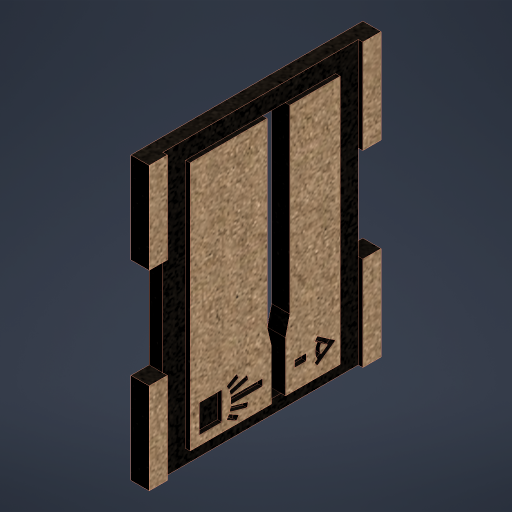
# Autodesk Inventor part: LightGate_Door_V1
Saved by Autodesk Inventor 2024.1 (Build 281209000, 209)
## iProperties
Created: 2023-05-21
Part Number: LightGate_Door_V1
Material: MDF Medium Density Fiberboard
Document SubType Name: Modeling
Designer: jaege
Density: 0.8 g/cm^3
Appearance: Red Oak - Natural Low Gloss
Mass: 15.6006 g
Surface Area: 117.953 cm^2
Volume: 19.5007 cm^3
Author: jaege
Autodesk Inventor part; units mm, degrees
ref_plane "YZ Plane" through (0, 0, 0) normal (1, 0, 0) x (0, 1, 0)
ref_plane "XZ Plane" through (0, 0, 0) normal (0, 1, 0) x (-1, 0, 0)
ref_plane "XY Plane" through (0, 0, 0) normal (0, 0, 1) x (1, 0, 0)
sketch "Sketch1" plane through (0, 0, 0) normal (1, 0, 0) x (0, 1, 0)
  line L0 (-31, -23.5) -> (-10.3333, -23.5) construction
  line L1 (31, -23.5) -> (31, 23.5)
  line L2 (31, 23.5) -> (11, 23.5)
  line L3 (-31, 23.5) -> (-31, -23.5)
  line L4 (-31, -23.5) -> (31, 23.5) construction
  line L5 (31, -23.5) -> (-31, 23.5) construction
  line L6 (-11, 23.5) -> (-11, 19.5)
  line L7 (-11, 19.5) -> (11, 19.5)
  line L8 (11, 19.5) -> (11, 23.5)
  line L9 (11, 23.5) -> (-11, 23.5) construction
  line L10 (-11, 23.5) -> (-31, 23.5)
  line L11 (31, -23.5) -> (10.3333, -23.5) construction
  line L12 (10.3333, -23.5) -> (10.3333, -27.5)
  line L13 (10.3333, -27.5) -> (31, -27.5)
  line L14 (31, -27.5) -> (31, -23.5)
  line L15 (-31, -23.5) -> (-10.3333, -23.5) construction
  line L16 (-10.3333, -23.5) -> (-10.3333, -27.5)
  line L17 (-10.3333, -27.5) -> (-31, -27.5)
  line L18 (-31, -27.5) -> (-31, -23.5)
  line L19 (10.3333, -23.5) -> (31, -23.5) construction
  line L20 (-10.3333, -23.5) -> (10.3333, -23.5)
  point P0 (0, 0)
  point P1 (11, 21.5)
  dimension "d0" = 62
  dimension "d1" = 47
  dimension "d2" = 20
  dimension "d3" = 4
  dimension "d5" = 4
  constraints: 42 end point, 13 parallel, 4 horizontal, 4 perpendicular, 3 equal length, 3 midpoint, 1 collinear, 1 horizontal alignment, 1 vertical
  measures "d0" distance of L3.start L1.end
  measures "d1" distance of L1.end L1.start
  measures "d2" distance from line of L1 point (11, 21.5)
  measures "d3" distance between parallel lines of L9 L7
  measures "d5" distance of L12.end L11.end
extrude "Outline" add sketch "Sketch1" along normal blind 4
sketch "Sketch2" plane through (4, 0, 0) normal (1, 0, 0) x (0, 0, -1)
  line L0 (3.4, 27) -> (3.4, -27.9)
  line L1 (3.4, -27.9) -> (6.5, -27.9)
  line L2 (6.5, -27.9) -> (6.5, 27)
  line L3 (6.5, 27) -> (3.4, 27)
  line L4 (-14.5, -0.45) -> (-5.55, -0.45) construction
  line L5 (-5.55, -0.45) -> (3.4, -0.45) construction
  line L6 (18.5, -0.45) -> (6.5, -0.45) construction
  line L7 (-19.5, 31) -> (23.5, 31)
  line L8 (23.5, 31) -> (23.5, -31)
  line L9 (-19.5, -31) -> (-19.5, 31)
  line L10 (-14.5, 27) -> (18.5, 27)
  line L11 (18.5, 27) -> (18.5, -27.9)
  line L12 (18.5, -27.9) -> (-14.5, -27.9)
  line L13 (-14.5, -27.9) -> (-14.5, 27)
  line L14 (-12.5, -19.7) -> (-7.5, -19.7)
  line L15 (-7.5, -19.7) -> (-7.5, -25.9)
  line L16 (-7.5, -25.9) -> (-12.5, -25.9)
  line L17 (-12.5, -25.9) -> (-12.5, -19.7)
  line L18 (-5.5, -22.05) -> (1.4, -22.05)
  line L19 (1.4, -22.05) -> (1.4, -23.55)
  line L20 (1.4, -23.55) -> (-5.5, -23.55)
  line L21 (-5.5, -23.55) -> (-5.5, -22.05)
  line L22 (13.4738, -19.9808) -> (17.5, -22.8)
  line L23 (17.5, -22.8) -> (13.4738, -25.6192)
  line L24 (13.4738, -19.9808) -> (12.9003, -20.8)
  line L25 (12.9003, -20.8) -> (15.7566, -22.8)
  line L26 (15.7566, -22.8) -> (12.9003, -24.8)
  line L27 (12.9003, -24.8) -> (13.4738, -25.6192)
  line L28 (-12.5, -22.8) -> (15.7566, -22.8) construction
  arc A0 (13.5039, -21.2227) -> (13.5039, -24.3773) centre (15.7566, -22.8) ccw
  arc A1 (14.323, -21.7962) -> (14.323, -23.8038) centre (15.7566, -22.8) ccw
  line L29 (8.5, -22.05) -> (11.0066, -22.05)
  line L30 (11.0066, -22.05) -> (11.0066, -23.55)
  line L31 (11.0066, -23.55) -> (8.5, -23.55)
  line L32 (8.5, -23.55) -> (8.5, -22.05)
  line L33 (-5.8236, -20.7956) -> (-5.548, -21.7568)
  line L34 (-5.548, -21.7568) -> (-1.703, -20.6543)
  line L35 (-1.703, -20.6543) -> (-1.9786, -19.693)
  line L36 (-1.9786, -19.693) -> (-5.8236, -20.7956)
  line L37 (-5.548, -23.8432) -> (-1.703, -24.9457)
  line L38 (-1.703, -24.9457) -> (-1.9786, -25.907)
  line L39 (-1.9786, -25.907) -> (-5.8236, -24.8044)
  line L40 (-5.8236, -24.8044) -> (-5.548, -23.8432)
  circle A2 centre (-11, -22.8) radius 5.5509 construction
  line L41 (-6.4623, -19.6028) -> (-5.9623, -20.4688)
  line L42 (-5.9623, -20.4688) -> (-3.7973, -19.2188)
  line L43 (-3.7973, -19.2188) -> (-4.2973, -18.3528)
  line L44 (-4.2973, -18.3528) -> (-6.4623, -19.6028)
  line L45 (-5.9623, -25.1312) -> (-6.4623, -25.9972)
  line L46 (-6.4623, -25.9972) -> (-4.2973, -27.2472)
  line L47 (-4.2973, -27.2472) -> (-3.7973, -26.3812)
  line L48 (-3.7973, -26.3812) -> (-5.9623, -25.1312)
  line L49 (23.5, 10.3333) -> (27.5, 10.3333) projected
  line L50 (27.5, 10.3333) -> (27.5, 31) projected
  line L51 (27.5, 31) -> (-23.5, 31) projected
  line L52 (-23.5, 31) -> (-23.5, 11) projected
  line L53 (-23.5, 11) -> (-19.5, 11) projected
  line L54 (-19.5, 11) -> (-19.5, -11) projected
  line L55 (-19.5, -11) -> (-23.5, -11) projected
  line L56 (-23.5, -11) -> (-23.5, -31) projected
  line L57 (-23.5, -31) -> (27.5, -31) projected
  line L58 (27.5, -31) -> (27.5, -10.3333) projected
  line L59 (27.5, -10.3333) -> (23.5, -10.3333) projected
  line L60 (23.5, -10.3333) -> (23.5, 10.3333) projected
  point P0 (0, 0)
  point P1 (-7.5, -22.8)
  point P2 (-5.5, -22.8)
  point P3 (13.0066, -22.8)
  point P4 (6.5, 27)
  point P5 (3.4, 27)
  dimension "d14" = 3.1
  dimension "d17" = 5
  dimension "d19" = 5
  dimension "d22" = 35
  dimension "d23" = 35
  dimension "d24" = 4
  dimension "d25" = 1
  dimension "d26" = 1
  dimension "d27" = 2.75
  dimension "d29" = 1
  dimension "d30" = 1.5
  dimension "d31" = 2
  dimension "d32" = 2
  dimension "d33" = 2
  dimension "d34" = 2
  dimension "d35" = 2
  dimension "d36" = 5
  dimension "d37" = 2
  dimension "d38" = 1
  dimension "d39" = 1
  dimension "d42" = 3.5
  dimension "d43" = 16
  dimension "d44" = 16
  dimension "d45" = 4
  dimension "d47" = 2.5
  dimension "d48" = 1
  dimension "d49" = 14
  dimension "d50" = 14
  dimension "d51" = 1
  dimension "d52" = 2.5
  dimension "d62" = 12
  dimension "d65" = 6.2
  dimension "d66" = 4
  dimension "d67" = 3.1
  constraints: 98 end point, 19 parallel, 15 perpendicular, 7 horizontal, 7 midpoint, 7 point on line, 5 point on circle, 4 collinear, 4 horizontal alignment, 3 vertical alignment, 2 centre point, 2 equal length, 1 concentric, 1 vertical, 11 other
  measures "d14" distance between parallel lines of L2 L0
  measures "d17" distance between parallel lines of L9 L13
  measures "d19" distance between parallel lines of L8 L11
  measures "d22" angle of L22 L28
  measures "d23" angle of L23 L28
  measures "d24" distance of L26.end L24.end
  measures "d25" radial gap between concentric circles of A1 A0
  measures "d26" distance between parallel lines of L22 L25
  measures "d27" radius of A0
  measures "d29" distance from line of L11 L22.end
  measures "d30" distance of L20.end L18.start
  measures "d31" distance between parallel lines of L0 L19
  measures "d32" distance between parallel lines of L2 L32
  measures "d33" distance from line of point (13.007, -22.8) L30
  measures "d34" distance between parallel lines of L13 L17
  measures "d35" distance between parallel lines of L12 L16
  measures "d36" distance between parallel lines of L17 L15
  measures "d37" distance between parallel lines of L15 L21
  measures "d38" distance of L34.end L35.end
  measures "d39" distance of L37.end L38.end
  measures "d42" distance from line of L15 point (-11, -22.8)
  measures "d43" angle of L37 L20
  measures "d44" angle of L34 L18
  measures "d45" distance of L35.end L33.start
  measures "d47" distance of L42.end L41.end
  measures "d48" distance of L42.end L43.end
  measures "d49" angle of L36 L42
  measures "d50" angle of L39 L48
  measures "d51" distance of L46.end L47.end
  measures "d52" distance of L47.end L45.start
  measures "d62" distance of L6.start L6.end
  measures "d65" distance of L16.end L14.start
  measures "d66" distance between parallel lines of L7 L10
  measures "d67" distance between parallel lines of L57 L12
extrude "Engravings" cut sketch "Sketch2" against normal blind 1 contours L3 L2 L1 L0 | L7 L8 L57 L9 | L14 L15 L16 L17 | L18 L19 L20 L21 | L22 L23 L27 L26 L25 L24 | L25 A1 L26 A0 | L29 L30 L31 L32 | L36 L35 L34 L33 | L37 L38 L39 L40 | L44 L43 L42 L41 | L48 L47 L46 L45
sketch "Sketch3" plane through (4, 0, 0) normal (1, 0, 0) x (0, 0, -1)
  line L0 (-7.5, -19.7) -> (-7.5, -25.9) projected
  line L1 (-7.5, -25.9) -> (-12.5, -25.9) projected
  line L2 (-12.5, -25.9) -> (-12.5, -19.7) projected
  line L3 (-12.5, -19.7) -> (-7.5, -19.7) projected
  line L4 (-3.7973, -26.3812) -> (-4.2973, -27.2472) projected
  line L5 (-4.2973, -27.2472) -> (-6.4623, -25.9972) projected
  line L6 (-6.4623, -25.9972) -> (-5.9623, -25.1312) projected
  line L7 (-5.9623, -25.1312) -> (-3.7973, -26.3812) projected
  line L8 (1.4, -22.05) -> (1.4, -23.55)
  line L9 (1.4, -23.55) -> (-5.5, -23.55) projected
  line L10 (-5.5, -23.55) -> (-5.5, -22.05) projected
  line L11 (-5.5, -22.05) -> (1.4, -22.05) projected
  line L12 (-4.2973, -18.3528) -> (-3.7973, -19.2188) projected
  line L13 (-3.7973, -19.2188) -> (-5.9623, -20.4688) projected
  line L14 (-5.9623, -20.4688) -> (-6.4623, -19.6028) projected
  line L15 (-6.4623, -19.6028) -> (-4.2973, -18.3528) projected
  line L16 (-1.9786, -19.693) -> (-1.703, -20.6543) projected
  line L17 (-1.703, -20.6543) -> (-5.548, -21.7568) projected
  line L18 (-5.548, -21.7568) -> (-5.8236, -20.7956) projected
  line L19 (-5.8236, -20.7956) -> (-1.9786, -19.693) projected
  line L20 (-1.703, -24.9457) -> (-1.9786, -25.907) projected
  line L21 (-1.9786, -25.907) -> (-5.8236, -24.8044) projected
  line L22 (-5.8236, -24.8044) -> (-5.548, -23.8432) projected
  line L23 (-5.548, -23.8432) -> (-1.703, -24.9457) projected
  line L24 (23.5, -31) -> (-19.5, -31) projected
  line L25 (23.5, 31) -> (23.5, 10.3333) projected
  line L26 (-19.5, 31) -> (23.5, 31) projected
  line L27 (-19.5, -11) -> (-19.5, 11) projected
  line L28 (18.5, -27.9) -> (18.5, 27) projected
  line L29 (-14.5, 27) -> (-14.5, -27.9) projected
  line L30 (3.4, -27.9) -> (6.5, -27.9)
  line L31 (2.45, 27) -> (2.45, -12.8)
  line L32 (2.45, -12.8) -> (3.4, -16.8)
  line L33 (7.45, 27) -> (7.45, -12.8)
  line L34 (7.45, -12.8) -> (6.5, -16.8)
  line L35 (6.5, -16.8) -> (6.5, -27.9)
  line L36 (-19.5, -31) -> (-19.5, -11) projected
  line L37 (23.5, 10.3333) -> (23.5, -10.3333) projected
  line L38 (-19.5, 11) -> (-19.5, 31) projected
  line L39 (23.5, -10.3333) -> (27.5, -10.3333) projected
  line L40 (27.5, -10.3333) -> (27.5, -31) projected
  line L41 (-14.5, -27.9) -> (18.5, -27.9) projected
  line L42 (3.4, -27.9) -> (3.4, 27) construction
  line L43 (6.5, 27) -> (6.5, -27.9) construction
  line L44 (18.5, 27) -> (6.5, 27) projected
  line L45 (3.4, 27) -> (-14.5, 27) projected
  line L46 (3.4, 27) -> (6.5, 27)
  line L47 (3.4, -27.9) -> (3.4, 27) construction
  line L48 (3.4, -16.8) -> (3.4, -27.9)
  point P0 (0, 0)
  dimension "d68" = 5
  dimension "d69" = 11.1
  dimension "d70" = 4
  constraints: 18 end point, 5 horizontal alignment, 2 vertical, 1 collinear, 1 equal length, 1 perpendicular, 1 vertical alignment
  measures "d68" distance between parallel lines of L33 L31
  measures "d69" distance of L34.end L30.end
  measures "d70" vertical distance of L34.end L33.end
extrude "Groove" cut sketch "Sketch3" against normal up to next contours L30 L48 L32 L31 L45 L46 L44 L33 L34 L35
sketch "Sketch4" plane through (3, 0, 0) normal (1, 0, 0) x (0, 0, -1)
  line L0 (-7.5, -25.9) -> (-7.5, -19.7) projected
  line L1 (-7.5, -19.7) -> (-12.5, -19.7) projected
  line L2 (-12.5, -19.7) -> (-12.5, -25.9) projected
  line L3 (-12.5, -25.9) -> (-7.5, -25.9) projected
  line L4 (-4.2973, -27.2472) -> (-3.7973, -26.3812) projected
  line L5 (-3.7973, -26.3812) -> (-5.9623, -25.1312) projected
  line L6 (-5.9623, -25.1312) -> (-6.4623, -25.9972) projected
  line L7 (-6.4623, -25.9972) -> (-4.2973, -27.2472) projected
  line L8 (14.323, -21.7962) -> (15.7566, -22.8) projected
  line L9 (15.7566, -22.8) -> (14.323, -23.8038) projected
  arc A0 (14.323, -21.7962) -> (14.323, -23.8038) centre (15.7566, -22.8) ccw projected
  line L10 (13.4738, -25.6192) -> (17.5, -22.8) projected
  line L11 (17.5, -22.8) -> (13.4738, -19.9808) projected
  line L12 (13.4738, -19.9808) -> (12.9003, -20.8) projected
  line L13 (12.9003, -20.8) -> (13.5039, -21.2227) projected
  arc A1 (13.5039, -21.2227) -> (13.5039, -24.3773) centre (15.7566, -22.8) ccw projected
  line L14 (13.5039, -24.3773) -> (12.9003, -24.8) projected
  line L15 (12.9003, -24.8) -> (13.4738, -25.6192) projected
  line L16 (1.4, -23.55) -> (1.4, -22.05) projected
  line L17 (1.4, -22.05) -> (-5.5, -22.05) projected
  line L18 (-5.5, -22.05) -> (-5.5, -23.55) projected
  line L19 (-5.5, -23.55) -> (1.4, -23.55) projected
  line L20 (27.5, 10.3333) -> (23.5, 10.3333) projected
  line L21 (27.5, 31) -> (27.5, 10.3333) projected
  line L22 (-23.5, 31) -> (-19.5, 31) projected
  line L23 (-19.5, -31) -> (-23.5, -31) projected
  line L24 (-23.5, 11) -> (-23.5, 31) projected
  line L25 (-19.5, 11) -> (-23.5, 11) projected
  line L26 (-23.5, -31) -> (-23.5, -11) projected
  line L27 (-23.5, -11) -> (-19.5, -11) projected
  line L28 (-3.7973, -19.2188) -> (-4.2973, -18.3528) projected
  line L29 (-4.2973, -18.3528) -> (-6.4623, -19.6028) projected
  line L30 (-6.4623, -19.6028) -> (-5.9623, -20.4688) projected
  line L31 (-5.9623, -20.4688) -> (-3.7973, -19.2188) projected
  line L32 (11.0066, -23.55) -> (11.0066, -22.05) projected
  line L33 (11.0066, -22.05) -> (8.5, -22.05) projected
  line L34 (8.5, -22.05) -> (8.5, -23.55) projected
  line L35 (8.5, -23.55) -> (11.0066, -23.55) projected
  line L36 (-1.703, -20.6543) -> (-1.9786, -19.693) projected
  line L37 (-1.9786, -19.693) -> (-5.8236, -20.7956) projected
  line L38 (-5.8236, -20.7956) -> (-5.548, -21.7568) projected
  line L39 (-5.548, -21.7568) -> (-1.703, -20.6543) projected
  line L40 (-1.9786, -25.907) -> (-1.703, -24.9457) projected
  line L41 (-1.703, -24.9457) -> (-5.548, -23.8432) projected
  line L42 (-5.548, -23.8432) -> (-5.8236, -24.8044) projected
  line L43 (-5.8236, -24.8044) -> (-1.9786, -25.907) projected
  line L44 (18.5, 27) -> (18.5, -27.9) projected
  line L45 (-14.5, -27.9) -> (-14.5, 27) projected
  line L46 (3.4, -27.9) -> (-14.5, -27.9) projected
  line L47 (23.5, -31) -> (-19.5, -31) projected
  line L48 (-19.5, -11) -> (-19.5, -31) projected
  line L49 (-19.5, -11) -> (-19.5, 11) projected
  line L50 (-19.5, 31) -> (-19.5, 11) projected
  line L51 (-19.5, 31) -> (23.5, 31) projected
  line L52 (23.5, 10.3333) -> (23.5, 31) projected
  line L53 (23.5, 10.3333) -> (23.5, -10.3333) projected
  line L54 (23.5, 31) -> (27.5, 31) projected
  line L55 (-14.5, 27) -> (2.45, 27) projected
  line L56 (7.45, 27) -> (18.5, 27) projected
  line L57 (18.5, -27.9) -> (6.5, -27.9) projected
  line L58 (7.45, 27) -> (2.45, 27) projected
  line L59 (7.45, -12.8) -> (7.45, 27) projected
  line L60 (6.5, -16.8) -> (7.45, -12.8) projected
  line L61 (6.5, -27.9) -> (6.5, -16.8) projected
  line L62 (3.4, -16.8) -> (3.4, -27.9) projected
  line L63 (2.45, -12.8) -> (3.4, -16.8) projected
  line L64 (2.45, 27) -> (2.45, -12.8) projected
  line L65 (3.4, -27.9) -> (6.5, -27.9) projected
  line L66 (23.5, -31) -> (23.5, -10.3333) projected
  line L67 (27.5, -31) -> (23.5, -31) projected
  line L68 (27.5, -10.3333) -> (27.5, -31) projected
  line L69 (23.5, -10.3333) -> (27.5, -10.3333) projected
  point P0 (0, 0)
sketch "Sketch5" plane through (3, 0, 0) normal (1, 0, 0) x (0, 0, -1)
  line L0 (-1.9786, -25.907) -> (-1.703, -24.9457) projected
  line L1 (-1.703, -24.9457) -> (-5.548, -23.8432) projected
  line L2 (-5.548, -23.8432) -> (-5.8236, -24.8044) projected
  line L3 (-5.8236, -24.8044) -> (-1.9786, -25.907) projected
  line L4 (-7.5, -25.9) -> (-7.5, -19.7) projected
  line L5 (-7.5, -19.7) -> (-12.5, -19.7) projected
  line L6 (-12.5, -19.7) -> (-12.5, -25.9) projected
  line L7 (-12.5, -25.9) -> (-7.5, -25.9) projected
  line L8 (1.4, -23.55) -> (1.4, -22.05) projected
  line L9 (1.4, -22.05) -> (-5.5, -22.05) projected
  line L10 (-5.5, -22.05) -> (-5.5, -23.55) projected
  line L11 (-5.5, -23.55) -> (1.4, -23.55) projected
  line L12 (-4.2973, -27.2472) -> (-3.7973, -26.3812) projected
  line L13 (-3.7973, -26.3812) -> (-5.9623, -25.1312) projected
  line L14 (-5.9623, -25.1312) -> (-6.4623, -25.9972) projected
  line L15 (-6.4623, -25.9972) -> (-4.2973, -27.2472) projected
  line L16 (-14.5, -27.9) -> (-14.5, 27) projected
  line L17 (-14.5, 27) -> (2.45, 27) projected
  line L18 (7.45, 27) -> (2.45, 27) projected
  line L19 (7.45, -12.8) -> (7.45, 27) projected
  line L20 (6.5, -16.8) -> (7.45, -12.8) projected
  line L21 (6.5, -27.9) -> (6.5, -16.8) projected
  line L22 (3.4, -27.9) -> (6.5, -27.9) projected
  line L23 (3.4, -16.8) -> (3.4, -27.9) projected
  line L24 (2.45, -12.8) -> (3.4, -16.8) projected
  line L25 (2.45, 27) -> (2.45, -12.8) projected
  line L26 (3.4, -27.9) -> (-14.5, -27.9) projected
  line L27 (7.45, 27) -> (18.5, 27) projected
  line L28 (18.5, 27) -> (18.5, -27.9) projected
  line L29 (18.5, -27.9) -> (6.5, -27.9) projected
  line L30 (23.5, -31) -> (23.5, -10.3333) projected
  line L31 (23.5, 10.3333) -> (23.5, -10.3333) projected
  line L32 (23.5, 10.3333) -> (23.5, 31) projected
  line L33 (-19.5, 31) -> (23.5, 31) projected
  line L34 (-19.5, 31) -> (-19.5, 11) projected
  line L35 (-19.5, -11) -> (-19.5, 11) projected
  line L36 (-19.5, -11) -> (-19.5, -31) projected
  line L37 (23.5, -31) -> (-19.5, -31) projected
  line L38 (27.5, -31) -> (23.5, -31) projected
  line L39 (27.5, -10.3333) -> (27.5, -31) projected
  line L40 (23.5, -10.3333) -> (27.5, -10.3333) projected
  line L41 (27.5, 10.3333) -> (23.5, 10.3333) projected
  line L42 (27.5, 31) -> (27.5, 10.3333) projected
  line L43 (23.5, 31) -> (27.5, 31) projected
  line L44 (-23.5, 31) -> (-19.5, 31) projected
  line L45 (-23.5, 11) -> (-23.5, 31) projected
  line L46 (-19.5, 11) -> (-23.5, 11) projected
  line L47 (-23.5, -11) -> (-19.5, -11) projected
  line L48 (-23.5, -31) -> (-23.5, -11) projected
  line L49 (-19.5, -31) -> (-23.5, -31) projected
  line L50 (-1.703, -20.6543) -> (-1.9786, -19.693) projected
  line L51 (-1.9786, -19.693) -> (-5.8236, -20.7956) projected
  line L52 (-5.8236, -20.7956) -> (-5.548, -21.7568) projected
  line L53 (-5.548, -21.7568) -> (-1.703, -20.6543) projected
  line L54 (14.323, -21.7962) -> (15.7566, -22.8) projected
  line L55 (15.7566, -22.8) -> (14.323, -23.8038) projected
  arc A0 (14.323, -21.7962) -> (14.323, -23.8038) centre (15.7566, -22.8) ccw projected
  line L56 (13.4738, -25.6192) -> (17.5, -22.8) projected
  line L57 (17.5, -22.8) -> (13.4738, -19.9808) projected
  line L58 (13.4738, -19.9808) -> (12.9003, -20.8) projected
  line L59 (12.9003, -20.8) -> (13.5039, -21.2227) projected
  arc A1 (13.5039, -21.2227) -> (13.5039, -24.3773) centre (15.7566, -22.8) ccw projected
  line L60 (13.5039, -24.3773) -> (12.9003, -24.8) projected
  line L61 (12.9003, -24.8) -> (13.4738, -25.6192) projected
  line L62 (11.0066, -23.55) -> (11.0066, -22.05) projected
  line L63 (11.0066, -22.05) -> (8.5, -22.05) projected
  line L64 (8.5, -22.05) -> (8.5, -23.55) projected
  line L65 (8.5, -23.55) -> (11.0066, -23.55) projected
  line L66 (-3.7973, -19.2188) -> (-4.2973, -18.3528) projected
  line L67 (-4.2973, -18.3528) -> (-6.4623, -19.6028) projected
  line L68 (-6.4623, -19.6028) -> (-5.9623, -20.4688) projected
  line L69 (-5.9623, -20.4688) -> (-3.7973, -19.2188) projected
  point P0 (0, 0)
body "Solid1"
